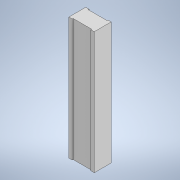
# Autodesk Inventor part: hook-coil I beam
Saved by Autodesk Inventor 2021 (Build 250183000, 183)
## iProperties
Created: 2021-04-24
Part Number: hook-coil I beam
Material: Generic
Document SubType Name: Modeling
Designer: newic
Density: 1 g/cm^3
Appearance: Default
Author: newic
Autodesk Inventor part; units mm, degrees
ref_plane "YZ Plane" through (0, 0, 0) normal (1, 0, 0) x (0, 1, 0)
ref_plane "XZ Plane" through (0, 0, 0) normal (0, 1, 0) x (-1, 0, 0)
ref_plane "XY Plane" through (0, 0, 0) normal (0, 0, 1) x (1, 0, 0)
sketch "Sketch1" plane through (0, 0, 0) normal (0, 1, 0) x (-1, 0, 0)
  line L0 (0, 0) -> (297.0107, 0) construction
  line L1 (297.0107, 0) -> (297.0107, -209.9733) construction
  line L2 (297.0107, -209.9733) -> (0, -209.9733) construction
  line L3 (0, -209.9733) -> (0, 0) construction
  line L4 (0, 0) -> (3.556, 0)
  line L5 (3.556, 0) -> (3.556, -17.526)
  line L6 (3.556, -17.526) -> (0, -17.526)
  line L7 (0, -17.526) -> (0, 0)
  line L8 (3.556, 0) -> (4.445, 0)
  line L9 (4.445, 0) -> (4.445, -0.889)
  line L10 (4.445, -0.889) -> (3.556, -0.889)
  line L11 (3.556, -0.889) -> (3.556, 0)
  line L12 (3.556, -17.526) -> (4.445, -17.526)
  line L13 (4.445, -17.526) -> (4.445, -16.637)
  line L14 (4.445, -16.637) -> (3.556, -16.637)
  line L15 (3.556, -16.637) -> (3.556, -17.526)
  line L16 (3.556, -0.889) -> (26.416, -0.889)
  line L17 (26.416, -0.889) -> (26.416, -16.637)
  line L18 (26.416, -16.637) -> (3.556, -16.637)
  line L19 (3.556, -16.637) -> (3.556, -0.889)
  line L20 (26.416, 0) -> (25.5359, 0)
  line L21 (25.5359, 0) -> (25.5359, -17.526)
  line L22 (25.5359, -17.526) -> (26.416, -17.526)
  line L23 (26.416, -17.526) -> (26.416, 0)
  line L24 (26.416, 0) -> (22.86, 0)
  line L25 (22.86, 0) -> (22.86, -17.526)
  line L26 (22.86, -17.526) -> (26.416, -17.526)
  line L27 (26.416, -17.526) -> (26.416, 0)
  point P0 (22.86, -0.889)
  point P1 (22.86, -16.637)
  dimension "d1" = 17.526
  dimension "d2" = 3.556
  dimension "d3" = 0.889
  dimension "d4" = 0.889
  dimension "d5" = 0.889
  dimension "d6" = 0.889
  dimension "d7" = 22.86
  dimension "d9" = 3.556
  constraints: 48 end point, 12 parallel, 6 horizontal, 6 perpendicular, 3 point on line, 2 other
  measures "d1" distance of L4.end L5.end
  measures "d2" distance of L5.end L6.end
  measures "d3" distance of L8.end L9.end
  measures "d4" distance of L14.end L13.end
  measures "d5" distance of L12.end L13.end
  measures "d6" distance of L9.end L10.end
  measures "d7" distance of L17.end L18.end
  measures "d9" distance of L26.end L25.end
extrude "Extrusion1" add sketch "Sketch1" along normal blind 127 contours L4 L5 L6 L7 | L10 L16 L25 L18 L14 L5 | L25 L24 L21 L16 | L16 L21 L18 L25 | L18 L21 L26 L25 | L21 L20 L23 L16 | L16 L17 L18 L21 | L18 L23 L22 L21
body "Solid1"
